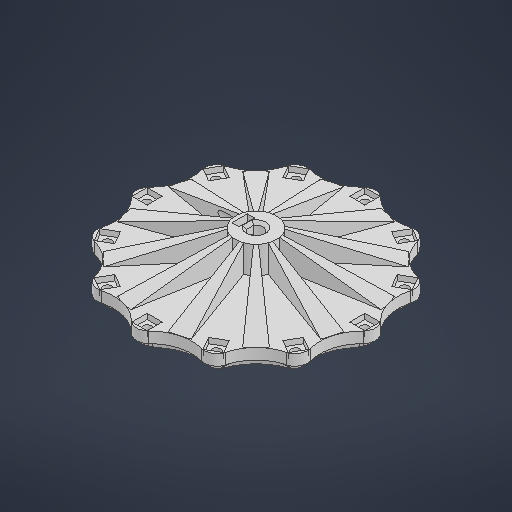
# Autodesk Inventor part: Shaft Collar
Saved by Autodesk Inventor 2025.1 (Build 291241000, 241)
## iProperties
Created: 2025-02-24
Part Number: Shaft Collar
Material: Generic
Document SubType Name: Modeling
Designer: jerem
Density: 1 g/cm^3
Appearance: Default
Author: jerem
## iProperties of the stored document Shaft Collar_3DPrint.ipt
Created: 2025-02-24
Part Number: Shaft Collar_3DPrint
Material: Generic
Document SubType Name: Modeling
Designer: jerem
Density: 1 g/cm^3
Appearance: Default
Author: jerem
Autodesk Inventor part; units mm, degrees
ref_plane "YZ Plane" through (0, 0, 0) normal (1, 0, 0) x (0, 1, 0)
ref_plane "XZ Plane" through (0, 0, 0) normal (0, 1, 0) x (-1, 0, 0)
ref_plane "XY Plane" through (0, 0, 0) normal (0, 0, 1) x (1, 0, 0)
sketch "Sketch1" plane through (0, 0, 0) normal (0, 1, 0) x (-1, 0, 0)
  circle A0 centre (0, 0) radius 2.6
  circle A1 centre (0, 0) radius 7.5
  circle A2 centre (0, 0) radius 39.75
  line L0 (2.2, 1.385641) -> (2.2, -1.385641)
  line L1 (2.2, 0) -> (-2.6, 0) construction
  line L2 (-40, 0) -> (-40, 0) construction
  circle A3 centre (-40, 0) radius 1.6
  line L3 (0, 0) -> (-38.395552, 10.288057)
  line L4 (-38.395552, 10.288057) -> (-53.367402, 14.299752) construction
  arc A4 (-42.530777, 3.217444) -> (-38.395552, 10.288057) centre (-53.367402, 14.299752) ccw
  line L5 (-40, 0) -> (-43.884659, 0) construction
  arc A5 (-42.530777, 3.217444) -> (-43.884659, 0) centre (-39.384659, 0) ccw
  line L6 (0, 0) -> (-38.395552, -10.288057)
  arc A6 (-38.395552, -10.288057) -> (-42.530777, -3.217444) centre (-53.367402, -14.299752) ccw
  arc A7 (-43.884659, 0) -> (-42.530777, -3.217444) centre (-39.384659, 0) ccw
  line L7 (-42.775, 2.775) -> (-37.225, 2.775)
  line L8 (-37.225, 2.775) -> (-37.225, -2.775)
  line L9 (-37.225, -2.775) -> (-42.775, -2.775)
  line L10 (-42.775, -2.775) -> (-42.775, 2.775)
  line L11 (-42.775, 2.775) -> (-37.225, -2.775) construction
  line L12 (-37.225, 2.775) -> (-42.775, -2.775) construction
  point P0 (-39.718781, 1.575092)
  point P1 (-39.718781, -1.575092)
  point P2 (-38.395552, -10.288057)
  point P3 (-38.395552, 10.288057)
  dimension "d0" = 5.2
  dimension "d3" = 15
  dimension "d4" = 79.5
  dimension "d21" = 3.2
  dimension "d23" = 40
  dimension "d45" = 15
  dimension "d46" = 31
  dimension "d48" = 39.75
  dimension "d49" = 4.5
  dimension "d70" = 5.55
  dimension "d73" = 4.8
  constraints: 26 end point, 11 point on circle, 8 centre point, 5 coincident, 3 horizontal, 3 midpoint, 3 perpendicular, 3 symmetric about line, 2 line through centre, 2 parallel, 1 collinear, 1 tangent, 1 vertical, 2 other
  measures "d0" diameter of A0
  measures "d3" diameter of A1
  measures "d4" diameter of A2
  measures "d21" diameter of A3
  measures "d23" distance of point (0, 0) L2.end
  measures "d45" angle of L1 L3
  measures "d46" diameter of A4
  measures "d48" distance of L3.end point (0, 0)
  measures "d49" radius of A5
  measures "d70" distance of L8.end L9.end
  measures "d73" distance of L1.end L1.start
extrude "Extrusion1" add sketch "Sketch1" along normal blind 3 contours A0 L0 | A0 L3 A1 L6 | A0 L6 A1 L3 | L3 A2 L6 A1 | A1 L6 A2 L9 L8 L7 L3 | L7 L8 L9 A2 A3 | A3 A2 picked at (-39.297687, 0)
extrude "Extrusion2" add sketch "Sketch1" along normal blind 10 from surface at 3 contours A0 L0 | A0 L3 A1 L6 | A0 L6 A1 L3
sketch "Sketch2" plane through (-2.2, 0, 1.385641) normal (1, 0, 0) x (0, 0, -1)
  line L0 (2.771281, 13) -> (0, 13)
  line L1 (2.771281, 13) -> (0, 13)
  line L2 (0, 0) -> (0, 13)
  line L3 (0, 0) -> (2.771281, 0)
  line L4 (2.771281, 0) -> (2.771281, 13)
  circle A0 centre (1.385641, 8) radius 1.6
  line L5 (1.385641, 8) -> (1.385641, 13) construction
  point P0 (1.385641, 0)
  dimension "d9" = 3.2
  dimension "d10" = 5
  constraints: 2 end point, 1 centre point, 1 midpoint
  measures "d9" diameter of A0
  measures "d10" distance of L5.start L5.end
extrude "Extrusion3" cut sketch "Sketch2" against normal through all contours A0 L4 | L4 A0 L2 | L2 A0
sketch "Sketch3" plane through (0, 13, 0) normal (0, 1, 0) x (1, 0, 0)
  line L0 (-2.2, 1.385641) -> (-2.2, -1.385641)
  arc A0 (-2.2, -1.385641) -> (-2.2, 1.385641) centre (0, 0) ccw
  circle A1 centre (0, 0) radius 7.5
  line L1 (-6, -2.825) -> (-3.4, -2.825)
  line L2 (-3.4, -2.825) -> (-3.4, 2.825)
  line L3 (-3.4, 2.825) -> (-6, 2.825)
  line L4 (-6, 2.825) -> (-6, -2.825)
  line L5 (-6, -2.825) -> (-3.4, 2.825) construction
  line L6 (-3.4, -2.825) -> (-6, 2.825) construction
  line L7 (-3.4, 0) -> (-2.2, 0) construction
  point P0 (-4.7, 0)
  dimension "d13" = 1.2
  dimension "d14" = 5.65
  dimension "d15" = 2.6
  constraints: 14 end point, 4 midpoint, 2 parallel, 2 perpendicular, 1 horizontal
  measures "d13" distance of L7.start L7.end
  measures "d14" distance of L1.end L2.end
  measures "d15" distance of L2.end L3.end
ref_plane "Work Plane2" through (0, 8, 0) normal (0, 1, 0) x (1, 0, 0)
extrude "Extrusion4" cut sketch "Sketch3" along normal blind 10 and the other way blind 3 from surface at -5 contours L4 L3 L2 L1
extrude "Extrusion5" cut sketch "Sketch1" along normal through all contours A3 A2 picked at (-39.297687, 0)
extrude "Extrusion7" add sketch "Sketch1" along normal up to surface (3 mm away) contours A2 L7 L10 L9 A6 A7 A5 A4 | A2 A3 L9 L10 L7
extrude "Extrusion11" cut sketch "Sketch1" against normal blind 2 from surface at 3 contours L7 L8 L9 A2 A3 | A2 A3 L9 L10 L7 | A3 A2 | A2 A3
pattern_circular "Circular Pattern1" count 12 over 360 about axis through (0, 0, 0) along (0, 1, 0) of "Extrusion5", "Extrusion7", "Extrusion11"
sketch "Sketch4" plane through (0, 3, 0) normal (0, 1, 0) x (1, 0, 0)
  circle A0 centre (0, -40) radius 1.562086
  circle A1 centre (-20, -34.641016) radius 1.067324
  circle A2 centre (0, 0) radius 7.5
  line L0 (0, -40) -> (0, 0)
  line L1 (0, 0) -> (-20, -34.641016)
  line L2 (-20, -34.641016) -> (0, -40)
  line L3 (-10, -37.320508) -> (0, 0)
  circle A3 centre (0, -40) radius 1.6
  circle A4 centre (-20, -34.641016) radius 1.6
  constraints: 8 end point, 2 centre point, 1 coincident, 1 midpoint, 1 perpendicular, 1 vertical
ref_plane "Work Plane3" through (-10, 3, 37.320508) normal (0.9659258, 0, 0.258819) x (0.258819, 0, -0.9659258)
sketch "Sketch5" plane through (-10, 3, 37.320508) normal (0.9659258, 0, 0.258819) x (0.258819, 0, -0.9659258)
  line L0 (31.137033, 0) -> (31.137033, 10)
  line L1 (46.536996, 0) -> (30.737071, 0)
  line L2 (52.752621, 0) -> (46.536996, 0)
  line L3 (66.435757, 0) -> (52.752621, 0)
  line L4 (70.98591, 0) -> (66.435757, 0)
  line L5 (78.885873, 0) -> (70.98591, 0)
  line L6 (80.551344, 0) -> (78.885873, 0)
  line L7 (80.551344, 0) -> (80.551344, 0)
  line L8 (78.885873, 0) -> (80.551344, 0)
  line L9 (70.98591, 0) -> (78.885873, 0)
  line L10 (66.435757, 0) -> (70.98591, 0)
  line L11 (52.752621, 0) -> (66.435757, 0)
  line L12 (46.536996, 0) -> (52.752621, 0)
  line L13 (30.737071, 0) -> (46.536996, 0)
  line L14 (24.521446, 0) -> (30.737071, 0)
  line L15 (10.838309, 0) -> (24.521446, 0)
  line L16 (6.288156, 0) -> (10.838309, 0)
  line L17 (-1.611807, 0) -> (6.288156, 0)
  line L18 (-3.277278, 0) -> (-1.611807, 0)
  line L19 (-3.277278, 0) -> (-3.277278, 0)
  line L20 (-1.611807, 0) -> (-3.277278, 0)
  line L21 (6.288156, 0) -> (-1.611807, 0)
  line L22 (10.838309, 0) -> (6.288156, 0)
  line L23 (24.521446, 0) -> (10.838309, 0)
  line L24 (30.737071, 0) -> (24.521446, 0)
  line L25 (31.137033, 0) -> (46.137033, 0)
  line L26 (31.137033, 10) -> (-1.112967, 0)
  line L27 (-1.112967, 0) -> (-3.277278, 0)
  line L28 (38.637033, -5.6) -> (38.637033, 12.6)
  point P0 (38.637033, -3)
  point P1 (26.684271, 0)
  point P2 (29.884271, 0)
  point P3 (8.752762, 0)
  point P4 (11.952762, 0)
  point P5 (-1.6, 0)
  point P6 (1.6, 0)
  point P7 (-1.6, 0)
  point P8 (1.6, 0)
  point P9 (8.752762, 0)
  point P10 (11.952762, 0)
  point P11 (26.684271, 0)
  point P12 (29.884271, 0)
  point P13 (47.389795, 0)
  point P14 (50.589795, 0)
  point P15 (65.321304, 0)
  point P16 (68.521304, 0)
  point P17 (75.674066, 0)
  point P18 (78.874066, 0)
  point P19 (75.674066, 0)
  point P20 (78.874066, 0)
  point P21 (50.589795, 0)
  point P22 (47.389795, 0)
  point P23 (68.521304, 0)
  point P24 (65.321304, 0)
  point P25 (31.137033, 0)
  constraints: 2 end point
revolve "Revolution1" add sketch "Sketch5" angle 10 mid plane about axis through (0, -10, 0) along (0, 1, 0)
pattern_circular "Circular Pattern2" count 12 over 360 about axis through (0, 0, 0) along (0, 1, 0) of "Revolution1"
ref_plane "Work Plane4" through (-7.5, 0, 0) normal (1, 0, 0) x (0, 0, -1)
sketch "Sketch7" plane through (-7.5, 0, 0) normal (1, 0, 0) x (0, 0, -1)
  circle A0 centre (0, 8) radius 1.6 projected
  circle A1 centre (0, 8) radius 3
  point P0 (0, 0)
  dimension "d57" = 6
  constraints: 1 centre point, 1 coincident
  measures "d57" diameter of A1
extrude "Extrusion8" cut sketch "Sketch7" against normal through all contours A0 | A1
sketch "Sketch8" plane through (0, 0, 0) normal (0, -1, 0) x (1, 0, 0)
  circle A0 centre (34.641016, 20) radius 1.6
  circle A1 centre (20, 34.641016) radius 1.6
  circle A2 centre (0, 40) radius 1.6
  circle A3 centre (-20, 34.641016) radius 1.6
  circle A4 centre (-34.641016, 20) radius 1.6
  circle A5 centre (-40, 0) radius 1.6
  circle A6 centre (-34.641016, -20) radius 1.6
  circle A7 centre (-20, -34.641016) radius 1.6
  circle A8 centre (0, -40) radius 1.6
  circle A9 centre (20, -34.641016) radius 1.6
  circle A10 centre (34.641016, -20) radius 1.6
  arc A11 (38.441455, 18.479) -> (42.530777, 3.217444) centre (53.367402, 14.299752) ccw
  arc A12 (38.441455, 18.479) -> (35.224011, 24.051777) centre (34.108116, 19.69233) ccw
  arc A13 (24.051777, 35.224011) -> (35.224011, 24.051777) centre (39.06765, 39.06765) ccw
  arc A14 (24.051777, 35.224011) -> (18.479, 38.441455) centre (19.69233, 34.108116) ccw
  arc A15 (3.217444, 42.530777) -> (18.479, 38.441455) centre (14.299752, 53.367402) ccw
  arc A16 (3.217444, 42.530777) -> (-3.217444, 42.530777) centre (0, 39.384659) ccw
  arc A17 (-18.479, 38.441455) -> (-3.217444, 42.530777) centre (-14.299752, 53.367402) ccw
  arc A18 (-18.479, 38.441455) -> (-24.051777, 35.224011) centre (-19.69233, 34.108116) ccw
  arc A19 (-35.224011, 24.051777) -> (-24.051777, 35.224011) centre (-39.06765, 39.06765) ccw
  arc A20 (-35.224011, 24.051777) -> (-38.441455, 18.479) centre (-34.108116, 19.69233) ccw
  arc A21 (-42.530777, 3.217444) -> (-38.441455, 18.479) centre (-53.367402, 14.299752) ccw
  arc A22 (-42.530777, 3.217444) -> (-42.530777, -3.217444) centre (-39.384659, 0) ccw
  arc A23 (-38.441455, -18.479) -> (-42.530777, -3.217444) centre (-53.367402, -14.299752) ccw
  arc A24 (-38.441455, -18.479) -> (-35.224011, -24.051777) centre (-34.108116, -19.69233) ccw
  arc A25 (-24.051777, -35.224011) -> (-35.224011, -24.051777) centre (-39.06765, -39.06765) ccw
  arc A26 (-24.051777, -35.224011) -> (-18.479, -38.441455) centre (-19.69233, -34.108116) ccw
  arc A27 (-3.217444, -42.530777) -> (-18.479, -38.441455) centre (-14.299752, -53.367402) ccw
  arc A28 (-3.217444, -42.530777) -> (3.217444, -42.530777) centre (0, -39.384659) ccw
  arc A29 (18.479, -38.441455) -> (3.217444, -42.530777) centre (14.299752, -53.367402) ccw
  arc A30 (18.479, -38.441455) -> (24.051777, -35.224011) centre (19.69233, -34.108116) ccw
  arc A31 (35.224011, -24.051777) -> (24.051777, -35.224011) centre (39.06765, -39.06765) ccw
  arc A32 (35.224011, -24.051777) -> (38.441455, -18.479) centre (34.108116, -19.69233) ccw
  arc A33 (42.530777, -3.217444) -> (38.441455, -18.479) centre (53.367402, -14.299752) ccw
  arc A34 (42.530777, -3.217444) -> (42.530777, 3.217444) centre (39.384659, 0) ccw
  circle A35 centre (40, 0) radius 1.6
  line L0 (-2.2, 1.385641) -> (-2.2, -1.385641)
  arc A36 (-2.2, -1.385641) -> (-2.2, 1.385641) centre (0, 0) ccw
extrude "Extrusion9" add sketch "Sketch8" along normal blind 5
chamfer "Chamfer2" distance 4 angle 45 24 edges at (28.1075, -5, -28.1075) (38.0052, -5, -21.9423) (38.3956, -5, -10.2881) (43.8847, -5, 0) (38.3956, -5, 10.2881) (38.0052, -5, 21.9423) (28.1075, -5, 28.1075) (21.9423, -5, 38.0052) (10.2881, -5, 38.3956) (0, -5, 43.8847) (-10.2881, -5, 38.3956) (-21.9423, -5, 38.0052) (-28.1075, -5, 28.1075) (-38.0052, -5, 21.9423) (-38.3956, -5, 10.2881) (-43.8847, -5, 0) (-38.3956, -5, -10.2881) (-38.0052, -5, -21.9423) (-28.1075, -5, -28.1075) (-21.9423, -5, -38.0052) (-10.2881, -5, -38.3956) (0, -5, -43.8847) (10.2881, -5, -38.3956) (21.9423, -5, -38.0052)
sketch "Sketch9" plane through (0, -5, 0) normal (0, -1, 0) x (1, 0, 0)
  circle A0 centre (-10, 0) radius 1.7
  circle A1 centre (10, 0) radius 1.7
  line L0 (-10, 0) -> (10, 0) construction
  point P0 (0, 0)
  point P1 (0, 0)
  dimension "d65" = 3.4
  dimension "d66" = 3.4
  dimension "d67" = 20
  constraints: 2 centre point, 2 end point, 1 coincident, 1 horizontal, 1 midpoint
  measures "d65" diameter of A0
  measures "d66" diameter of A1
  measures "d67" distance of L0.start L0.end
extrude "Extrusion10" cut sketch "Sketch9" against normal blind 8
chamfer "Chamfer3" distance 1 angle 45 2 edges at (2.6, 13, 0) (-2.2, 13, 0)
equation "\"d48\" = 0.5 * d4"
body "Solid1"
